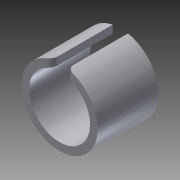
# Autodesk Inventor part: Aluminum Spacer Part 1
Saved by Autodesk Inventor 2013 (Build 170138000, 138)
## iProperties
Created: 2013-03-11
Part Number: Aluminum Spacer Part 1
Material: Aluminum 6061
Document SubType Name: Modeling
Designer: Moses
Density: 2.71 g/cm^3
Mass: 2.45241 g
Surface Area: 12.826 cm^2
Volume: 0.904948 cm^3
Author: Moses
Autodesk Inventor part; units mm, degrees
ref_plane "YZ Plane" through (0, 0, 0) normal (1, 0, 0) x (0, 1, 0)
ref_plane "XZ Plane" through (0, 0, 0) normal (0, 1, 0) x (-1, 0, 0)
ref_plane "XY Plane" through (0, 0, 0) normal (0, 0, 1) x (1, 0, 0)
sketch "Sketch1" plane through (0, 0, 0) normal (0, 0, 1) x (1, 0, 0)
  circle A0 centre (0, 0) radius 6.35
  circle A1 centre (0, 0) radius 7.9375
  line L0 (-1.5875, 7.7771) -> (-1.5875, 6.1484)
  line L1 (1.5875, 6.1484) -> (1.5875, 7.7771)
  line L2 (0, 0) -> (0, 7.9375) construction
  dimension "d0" = 12.7
  dimension "d1" = 15.875
  dimension "d4" = 1.5875
  dimension "d5" = 1.5875
  constraints: 6 end point, 5 point on circle, 2 centre point, 2 coincident, 1 parallel, 1 vertical
  measures "d0" diameter of A0
  measures "d1" diameter of A1
  measures "d4" distance between parallel lines of L2 L0
  measures "d5" distance between parallel lines of L1 L2
extrude "Extrusion1" add sketch "Sketch1" along normal blind 12.7 contours A0 L1 A1 L0 picked at (7.3341, -0.6223)
fillet "Fillet1" radius 1.27 2 edges at (-1.5875, 6.9627, 12.7) (1.5875, 6.9627, 12.7)
body "Solid1"
